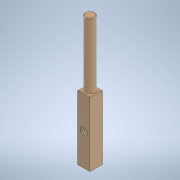
# Autodesk Inventor part: Ball Track Rest Pin
Saved by Autodesk Inventor 2021.1 (Build 251245010, 245A)
## iProperties
Created: 2025-09-16
Material: Bronze, Soft Tin
Document SubType Name: Modeling
Designer: SD
Density: 8.874 g/cm^3
Appearance: Brindle
Mass: 2.63132 g
Surface Area: 4.07665 cm^2
Volume: 0.29652 cm^3
Project: Automatic Tea Steeping mechanism
Part Number: Ball Track Rest Pin
Length: 42.000 mm
BOM-Mass: 0.00263
BOM-Area: 0.000
Square Bar: 4 mm x 4 mm
Author: SD
Title: Ball Track Rest Pin
Autodesk Inventor part; units mm, degrees
ref_plane "YZ Plane" through (0, 0, 0) normal (1, 0, 0) x (0, 1, 0)
ref_plane "XZ Plane" through (0, 0, 0) normal (0, 1, 0) x (-1, 0, 0)
ref_plane "XY Plane" through (0, 0, 0) normal (0, 0, 1) x (1, 0, 0)
sketch "Sketch4" plane through (0, 0, 0) normal (0, 1, 0) x (-1, 0, 0)
  circle A0 centre (0, 0) radius 1.5
  line L0 (-2, 2) -> (2, 2)
  line L1 (2, 2) -> (2, -2)
  line L2 (2, -2) -> (-2, -2)
  line L3 (-2, -2) -> (-2, 2)
  line L4 (-2, 2) -> (2, -2) construction
  line L5 (2, 2) -> (-2, -2) construction
  point P0 (-1.5, 0)
  point P1 (0, -1.5)
  point P2 (0, 1.5)
  point P3 (1.5, 0)
  dimension "Radius" = 3
  dimension "d103" = 4
  constraints: 12 end point, 2 midpoint, 2 parallel, 2 perpendicular, 1 centre point, 1 coincident, 1 horizontal
  measures "Radius" diameter of A0
  measures "d103" distance of L0.end L1.end
extrude "Extrusion2" add sketch "Sketch4" along normal mid plane 42 contours A0
extrude "Extrusion10" add sketch "Sketch4" against normal up to surface (21 mm away) contours A0 | L0 L1 L2 L3
chamfer "Chamfer1" distance 0.2 angle 45 9 edges at (1.5, 21, 0) (0, -21, -2) (2, -21, 0) (0, -21, 2) (-2, -21, 0) (2, 0, 0) (0, 0, 2) (-2, 0, 0) (0, 0, -2)
sketch "Sketch14" plane through (2, -0.2, -2) normal (0, 0, -1) x (-1, 0, 0)
  line L0 (0, 0) -> (0, -20.6) projected
  line L1 (0, -10.3) -> (2, -10.3) construction
  point P0 (2, 0.2)
  constraints: 2 end point, 1 coincident, 1 horizontal, 1 midpoint, 1 vertical alignment
hole "Hole6" at (0, -10.5, -2) direction (0, 0, 1) diameter 2.459 end through all thread size "M3x0.5" class "6H" standard "ISO Metric profile"
body "Solid2"
